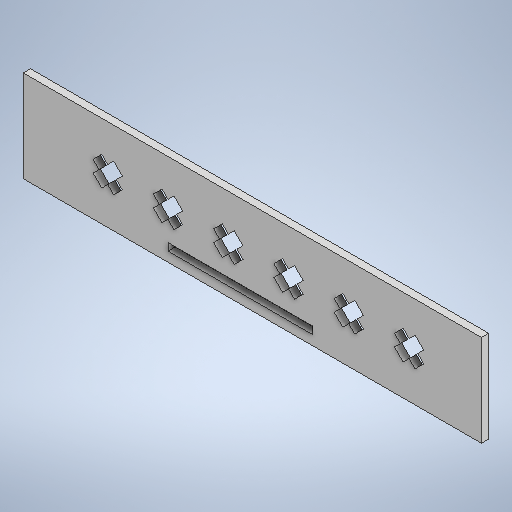
# Autodesk Inventor part: Extension.2
Saved by Autodesk Inventor 2025.4 (Build 294407000, 407)
## iProperties
Created: 2026-06-10
Part Number: Extension.2
Material: Generic
Document SubType Name: Sheet Metal
Designer: lenovo
Density: 1 g/cm^3
Sheet Metal Rule: Default_mm
Appearance: Default
Author: lenovo
Autodesk Inventor part; units mm, degrees
ref_plane "YZ Plane" through (0, 0, 0) normal (1, 0, 0) x (0, 1, 0)
ref_plane "XZ Plane" through (0, 0, 0) normal (0, 1, 0) x (-1, 0, 0)
ref_plane "XY Plane" through (0, 0, 0) normal (0, 0, 1) x (1, 0, 0)
sketch "Sketch1" plane through (0, 0, 0) normal (0, 0, 1) x (1, 0, 0)
  line L0 (-95, -19) -> (95, -19)
  line L1 (95, -19) -> (95, 19)
  line L2 (95, 19) -> (-95, 19)
  line L3 (-95, 19) -> (-95, -19)
  line L4 (-95, -19) -> (95, 19) construction
  line L5 (95, -19) -> (-95, 19) construction
  line L6 (-35, -11.92) -> (25, -11.92)
  line L7 (25, -11.92) -> (25, -15)
  line L8 (25, -15) -> (-35, -15)
  line L9 (-35, -15) -> (-35, -11.92)
  line L10 (-35, -11.92) -> (25, -15) construction
  line L11 (25, -11.92) -> (-35, -15) construction
  line L12 (62.5251, 6.067) -> (58.933, 2.4749)
  line L13 (58.933, 2.4749) -> (67.4749, -6.067)
  line L14 (67.4749, -6.067) -> (71.067, -2.4749)
  line L15 (71.067, -2.4749) -> (62.5251, 6.067)
  line L16 (67.4749, 6.067) -> (71.067, 2.4749)
  line L17 (71.067, 2.4749) -> (62.5251, -6.067)
  line L18 (62.5251, -6.067) -> (58.933, -2.4749)
  line L19 (58.933, -2.4749) -> (67.4749, 6.067)
  line L20 (60.7291, -4.2709) -> (69.2709, 4.2709)
  line L21 (60.7291, 4.2709) -> (69.2709, -4.2709)
  line L22 (0, 0) -> (95, 0)
  point P0 (-5, -13.46)
  point P1 (-5, -11.92)
  point P2 (65, 0)
  point P3 (68.5921, 0)
  point P4 (65, -3.5921)
  point P5 (61.4079, 0)
  point P6 (65, 3.5921)
  dimension "d0" = 38
  dimension "d1" = 190
  dimension "d2" = 3.08
  dimension "d3" = 60
  dimension "d4" = 100
  dimension "d5" = 4
  dimension "d6" = 45
  dimension "d7" = 5.08
  dimension "d8" = 12.08
  dimension "d9" = 30
  constraints: 46 end point, 12 midpoint, 9 parallel, 6 perpendicular, 2 horizontal, 1 horizontal alignment
  measures "d0" distance between parallel lines of L2 L0
  measures "d1" distance of L1.end L2.end
  measures "d2" distance between parallel lines of L6 L8
  measures "d3" distance of L6.start L6.end
  measures "d4" distance from line of L1 point (-5, -11.92)
  measures "d5" distance between parallel lines of L8 L0
  measures "d6" angle of L20 L22
  measures "d7" distance of L12.start L12.end
  measures "d8" distance of L16.end L17.end
  measures "d9" distance from line of L1 point (65, 0)
extrude "Plate1" add sketch "Sketch1" along normal blind 3 contours L15 L14 L21 L17 | L17 L21 L22 | L22 L20 L15 | L15 L20 L16 L17 | L3 L2 L1 L0 | L20 L21 L19 L15 | L15 L19 L16 L20 | L21 L14 L13 L17 | L17 L13 L20 L21 | L22 L19 L21 | L20 L13 L22 | L19 L21 L12 L15 | L17 L18 L20 L13 | L20 L18 L19 L13 | L19 L13 L12 L21
extrude "Cut1" cut sketch "Sketch1" along normal through all contours L15 L14 L21 L17 | L17 L21 L22 | L22 L20 L15 | L15 L20 L16 L17 | L20 L21 L19 L15 | L15 L19 L16 L20 | L21 L14 L13 L17 | L17 L13 L20 L21 | L22 L19 L21 | L20 L13 L22 | L19 L21 L12 L15 | L17 L18 L20 L13 | L20 L18 L19 L13 | L19 L13 L12 L21
pattern_linear "Rectangular Pattern1" count 6 spacing 25 along (-1, 0, 0) of "Cut1"
equation "\"d11\" = Thickness"
equation "\"d10\" = Thickness"
equation "\"BendRadius\" = Thickness"
equation "\"BendReliefWidth\" = Thickness"
equation "\"BendReliefDepth\" = 0.5 * Thickness"
equation "\"CornerReliefSize\" = 4 * Thickness"
equation "\"MinimumRemnant\" = 2 * Thickness"
equation "\"TransitionRadius\" = BendRadius"
equation "\"JacobiRadiusSize\" = BendRadius"
equation "\"GapSize\" = Thickness"
equation "\"Thickness\" = 3"
body "Solid1"
